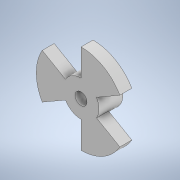
# Autodesk Inventor part: SlitDisc-FA130
Saved by Autodesk Inventor 2022 (Build 260153000, 153)
## iProperties
Created: 2024-07-04
Part Number: SlitDisc-FA130
Material: 一般
Document SubType Name: Modeling
Designer: yamashita1
Density: 1 g/cm^3
Appearance: 既定
Author: yamashita1
Autodesk Inventor part; units mm, degrees
ref_plane "YZ Plane" through (0, 0, 0) normal (1, 0, 0) x (0, 1, 0)
ref_plane "XZ Plane" through (0, 0, 0) normal (0, 1, 0) x (-1, 0, 0)
ref_plane "XY Plane" through (0, 0, 0) normal (0, 0, 1) x (1, 0, 0)
sketch "スケッチ1" plane through (0, 0, 0) normal (0, 0, 1) x (1, 0, 0)
  circle A0 centre (0, 0) radius 7.5
  dimension "DIA" = 15
  constraints: 1 centre point, 1 coincident
  measures "DIA" diameter of A0
extrude "押し出し1" add sketch "スケッチ1" along normal blind 2
sketch "スケッチ2" plane through (0, 0, 2) normal (0, 0, 1) x (1, 0, 0)
  line L0 (0, 0) -> (0, 15)
  line L1 (0, 0) -> (-12.9904, 7.5)
  line L2 (0, 0) -> (15, 0) construction
  line L3 (-12.9904, 7.5) -> (0, 15)
  circle A0 centre (0, 0) radius 3
  point P0 (-2.5981, 1.5)
  point P1 (0, 3)
  dimension "d3" = 15
  dimension "d4" = 15
  dimension "d5" = 150
  dimension "HUB_DIA" = 6
  constraints: 8 end point, 1 centre point, 1 coincident, 1 equal length, 1 horizontal, 1 vertical
  measures "d3" distance of L0.start L0.end
  measures "d4" distance of L0.start L1.end
  measures "d5" angle of L2 L1
  measures "HUB_DIA" diameter of A0
extrude "押し出し2" cut sketch "スケッチ2" against normal blind 2 contours A0 L1 L3 L0
pattern_circular "円形状パターン1" count 3 over 360 about axis through (0, 0, -10) along (0, 0, 1) of "押し出し2"
sketch "スケッチ3" plane through (0, 0, 0) normal (0, 0, -1) x (-1, 0, 0)
  circle A0 centre (0, 0) radius 3
  arc A1 (0, -3) -> (2.5981, -1.5) centre (0, 0) ccw projected
  constraints: 1 centre point, 1 coincident, 1 concentric
extrude "押し出し3" add sketch "スケッチ3" along normal blind 2
sketch "スケッチ4" plane through (0, 0, -2) normal (0, 0, -1) x (-1, 0, 0)
  point P0 (0, 0)
  point P1 (0, 0)
  constraints: 1 coincident
hole "穴1" at (0, 0, -2) direction (0, 0, 1) diameter 2 end through all
equation "\"d3\" = DIA"
equation "\"d4\" = DIA"
equation "\"d6\" = THIN"
equation "\"d12\" = THIN"
equation "\"THIN\" = 2"
